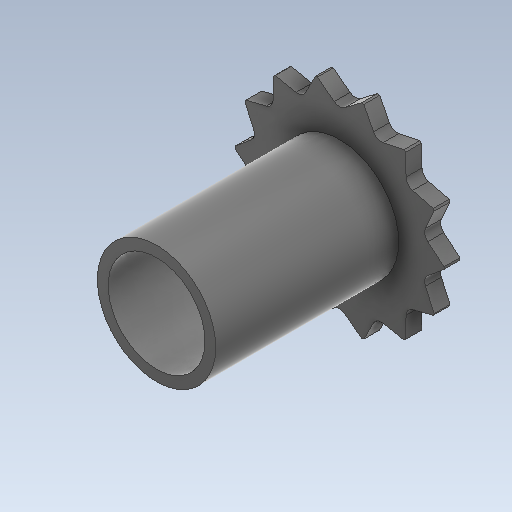
# Autodesk Inventor part: ВедущееКолесо
Saved by Autodesk Inventor 2020 (Build 240168000, 168)
## iProperties
Created: 2021-02-25
Part Number: ВедущееКолесо
Material: Пластик ЖКП
Document SubType Name: Modeling
Designer: I_Love_U_Bogdan
Density: 1.626 g/cm^3
Appearance: Гладкая — черная
Author: I_Love_U_Bogdan
Autodesk Inventor part; units mm, degrees
ref_plane "YZ Plane" through (0, 0, 0) normal (1, 0, 0) x (0, 1, 0)
ref_plane "XZ Plane" through (0, 0, 0) normal (0, 1, 0) x (-1, 0, 0)
ref_plane "XY Plane" through (0, 0, 0) normal (0, 0, 1) x (1, 0, 0)
sketch "Эскиз1" plane through (0, 0, 0) normal (0, 0, 1) x (1, 0, 0)
  circle A0 centre (0, 0) radius 22.47
  line L0 (21.9066, 5) -> (21.9066, -5)
  circle A1 centre (21.9066, -5) radius 2.05
  circle A2 centre (21.9066, 5) radius 2.05
  line L1 (21.9066, 5) -> (0, 0)
  line L2 (0, 0) -> (21.9066, -5)
  line L3 (21.9066, 5) -> (13.9325, -4.5032)
  circle A3 centre (0, 0) radius 15.4921
  line L4 (20.5889, 3.4296) -> (24.3782, 0.25)
  line L5 (0, 0) -> (4.0279, 0)
  line L6 (20.5889, -3.4296) -> (24.3782, -0.25)
  line L7 (24.3782, 0.25) -> (24.3782, -0.25)
  line L8 (21.9066, -5) -> (14.1251, 4.2737)
  line L9 (21.8556, 10.8026) -> (22.0725, 10.3521)
  circle A4 centre (21.9066, 5.0001) radius 2.05
  line L10 (20.038, 5.8432) -> (22.0725, 10.3521)
  line L11 (17.0619, 12.0232) -> (21.8556, 10.8026)
  circle A5 centre (17.5678, 14.0098) radius 2.05
  line L12 (15.0041, 19.2155) -> (15.395, 18.9038)
  circle A6 centre (17.5677, 14.0099) radius 2.05
  line L13 (15.5184, 13.9587) -> (15.395, 18.9038)
  line L14 (10.1556, 18.2354) -> (15.0041, 19.2155)
  circle A7 centre (9.7494, 20.2448) radius 2.05
  line L15 (5.1809, 23.8227) -> (5.6684, 23.7114)
  circle A8 centre (9.7493, 20.2448) radius 2.05
  line L16 (7.9251, 19.3096) -> (5.6684, 23.7114)
  line L17 (1.2378, 20.8359) -> (5.1809, 23.8227)
  circle A9 centre (0, 22.47) radius 2.05
  line L18 (-5.6684, 23.7114) -> (-5.1809, 23.8227)
  circle A10 centre (0, 22.47) radius 2.05
  line L19 (-1.2378, 20.8359) -> (-5.1809, 23.8227)
  line L20 (-7.9251, 19.3096) -> (-5.6684, 23.7114)
  circle A11 centre (-9.7493, 20.2448) radius 2.05
  line L21 (-15.395, 18.9038) -> (-15.0041, 19.2155)
  circle A12 centre (-9.7494, 20.2448) radius 2.05
  line L22 (-10.1556, 18.2354) -> (-15.0041, 19.2155)
  line L23 (-15.5184, 13.9587) -> (-15.395, 18.9038)
  circle A13 centre (-17.5677, 14.0099) radius 2.05
  line L24 (-22.0725, 10.3521) -> (-21.8556, 10.8026)
  circle A14 centre (-17.5678, 14.0098) radius 2.05
  line L25 (-17.0619, 12.0232) -> (-21.8556, 10.8026)
  line L26 (-20.038, 5.8432) -> (-22.0725, 10.3521)
  circle A15 centre (-21.9066, 5.0001) radius 2.05
  line L27 (-24.3782, -0.25) -> (-24.3782, 0.25)
  circle A16 centre (-21.9066, 5) radius 2.05
  line L28 (-20.5889, 3.4296) -> (-24.3782, 0.25)
  line L29 (-20.5889, -3.4296) -> (-24.3782, -0.25)
  circle A17 centre (-21.9066, -5) radius 2.05
  line L30 (-21.8556, -10.8026) -> (-22.0725, -10.3521)
  circle A18 centre (-21.9066, -5.0001) radius 2.05
  line L31 (-20.038, -5.8432) -> (-22.0725, -10.3521)
  line L32 (-17.0619, -12.0232) -> (-21.8556, -10.8026)
  circle A19 centre (-17.5678, -14.0098) radius 2.05
  line L33 (-15.0041, -19.2155) -> (-15.395, -18.9038)
  circle A20 centre (-17.5677, -14.0099) radius 2.05
  line L34 (-15.5184, -13.9587) -> (-15.395, -18.9038)
  line L35 (-10.1556, -18.2354) -> (-15.0041, -19.2155)
  circle A21 centre (-9.7494, -20.2448) radius 2.05
  line L36 (-5.1809, -23.8227) -> (-5.6684, -23.7114)
  circle A22 centre (-9.7493, -20.2448) radius 2.05
  line L37 (-7.9251, -19.3096) -> (-5.6684, -23.7114)
  line L38 (-1.2378, -20.8359) -> (-5.1809, -23.8227)
  circle A23 centre (0, -22.47) radius 2.05
  line L39 (5.6684, -23.7114) -> (5.1809, -23.8227)
  circle A24 centre (0, -22.47) radius 2.05
  line L40 (1.2378, -20.8359) -> (5.1809, -23.8227)
  line L41 (7.9251, -19.3096) -> (5.6684, -23.7114)
  circle A25 centre (9.7493, -20.2448) radius 2.05
  line L42 (15.395, -18.9038) -> (15.0041, -19.2155)
  circle A26 centre (9.7494, -20.2448) radius 2.05
  line L43 (10.1556, -18.2354) -> (15.0041, -19.2155)
  line L44 (15.5184, -13.9587) -> (15.395, -18.9038)
  circle A27 centre (17.5677, -14.0099) radius 2.05
  line L45 (22.0725, -10.3521) -> (21.8556, -10.8026)
  circle A28 centre (17.5678, -14.0098) radius 2.05
  line L46 (17.0619, -12.0232) -> (21.8556, -10.8026)
  line L47 (20.038, -5.8432) -> (22.0725, -10.3521)
  circle A29 centre (21.9066, -5.0001) radius 2.05
  line L48 (22.3878, 1.9202) -> (22.3878, -1.9202)
  circle A30 centre (0, 0) radius 11.3
  point P0 (21.9066, 0)
  point P1 (19.908, 4.5439)
  point P2 (15.965, 12.7317)
  point P3 (8.8599, 18.3978)
  point P4 (0, 20.42)
  point P5 (-8.8599, 18.3978)
  point P6 (-15.965, 12.7317)
  point P7 (-19.908, 4.5439)
  point P8 (-19.908, -4.5439)
  point P9 (-15.965, -12.7317)
  point P10 (-8.8599, -18.3978)
  point P11 (0, -20.42)
  point P12 (8.8599, -18.3978)
  point P13 (15.965, -12.7317)
  point P14 (19.908, -4.5439)
  point P15 (11.0167, -2.5145)
  point P16 (11.0167, 2.5145)
  point P17 (15.1037, 3.4473)
  point P18 (15.1037, -3.4473)
  dimension "d3" = 4.1
  dimension "d0" = 44.94
  dimension "d1" = 10
  dimension "d2" = 4.1
  dimension "d4" = 40
  dimension "d6" = 40
  dimension "d9" = 360
  dimension "d13" = 0.5
  dimension "d23" = 3.8403
  dimension "d24" = 22.6
  constraints: 98 end point, 17 centre point, 5 coincident, 4 point on circle, 3 point on line, 2 symmetric about line, 2 vertical, 1 horizontal, 1 midpoint, 1 perpendicular, 198 other
  measures "d0" diameter of A0
  measures "d1" distance of L0.start L0.end
  measures "d2" diameter of A1
  measures "d4" angle of L0 L3
  measures "d6" angle of L8 L0
  measures "d13" distance of L4.end L6.end
  measures "d23" distance of L48.start L48.end
  measures "d24" diameter of A30
extrude "Выдавливание1" add sketch "Эскиз1" along normal blind 3.7 contours A0 L48 | A0 L4 L7 L6 | L48 L6 L0 L4 | L0 L6 L8 L3 L4 | L3 L8 A3 L1 A2 | A1 L2 A3 L3 L8 | L1 A3 L2 A1 L47 A0 L46 A27 L44 L43 A25 L41 L40 A23 L38 L37 A21 L35 L34 A19 L32 L31 A17 L29 L28 A15 L26 L25 A13 L23 L22 A11 L20 L19 A9 L17 L16 A7 L14 L13 A5 L11 L10 A2 | L3 A3 L8 | A0 L11 L9 L10 | A3 L8 L1 | L1 A30 L2 A3 | A3 L2 L3 | L3 L2 A30 L1 L8 A3 | L47 L45 L46 A0 | A0 L14 L12 L13 | L44 L42 L43 A0 | A0 L17 L15 L16 | L41 L39 L40 A0 | A0 L20 L18 L19 | L38 L36 L37 A0 | A0 L23 L21 L22 | L35 L33 L34 A0 | A0 L26 L24 L25 | L32 L30 L31 A0 | A0 L29 L27 L28
sketch "Эскиз5" plane through (0, 0, 3.7) normal (0, 0, 1) x (1, 0, 0)
  circle A0 centre (0, 0) radius 13.8
  circle A1 centre (0, 0) radius 11.3 projected
  dimension "d25" = 2.5
  constraints: 1 centre point, 1 coincident
  measures "d25" radial gap between concentric circles of A1 A0
extrude "Выдавливание3" add sketch "Эскиз5" along normal blind 22.4
sketch "Эскиз6" plane through (0, 0, 26.1) normal (0, 0, 1) x (1, 0, 0)
  circle A0 centre (0, 0) radius 13.8
  circle A1 centre (-1.995, 7.7473) radius 1.55 projected
  circle A2 centre (7.7068, -2.1459) radius 1.55 projected
  circle A3 centre (-5.7118, -5.6014) radius 1.55 projected
  constraints: 1 centre point, 1 coincident
extrude "Выдавливание4" add sketch "Эскиз6" along normal blind 3
sketch "Эскиз7" plane through (0, 0, 29.1) normal (0, 0, 1) x (1, 0, 0)
  circle A0 centre (0, 0) radius 11.3 projected
  circle A1 centre (0, 0) radius 13.8 projected
extrude "Выдавливание5" add sketch "Эскиз7" along normal blind 17.3
equation "\"d2\" = d3"
